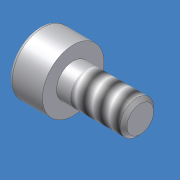
# Autodesk Inventor part: 520204172
Saved by Autodesk Inventor 2021.3 (Build 253353000, 353)
## iProperties
Manager: SRONS
Created: 2005-03-16
Part Number: 520204172
Material: Allgemein
Vendor: Autodesk Inc.
Document SubType Name: Modeling
Standard: DIN 912
Designer: SROAMA
Size Designation: M3 x 6
User Status: Zurückgezogen
Engineer: SROAMA
Density: 1 g/cm^3
Appearance: Vorgabe
Mass: 0.104143 g
Surface Area: 1.64552 cm^2
Volume: 0.104143 cm^3
Description: Zyl-Schr M3 x 6 DIN 912 A4 BN 612
Title: Zyl-Schr M3 x 6 DIN 912 A4 BN 612
Author: SROAMA
EGR: 1
Classification: un/spsc 31161501
Design Tracking - Titel: M3 x 6
Dateiname: 520_204_172
Zeichnungsummer: 520 204 172
Erstellt_am: 16.01.2008
Erstellt_durch: KC
Status: Veraltet
Titel: Zyl-Schr M3 x 6 ISO 4762 Inox A4
Zeichnungsname: 520 204 172
Zeichnungsnummer: 520204172
DOCID: 218911
PDB_IDENT: 520204172
PDB_Name: 520204172
PDB_Ident_Ver: =<PDB_Ident> <PDB_Version>
STID: 28675
ROT_Weight: 0.104 g
ROT_Weight_Num: 0.00010414301452605634
_DisabledCommands: 0
Autodesk Inventor part; units mm, degrees
ref_plane "YZ Plane" through (0, 0, 0) normal (1, 0, 0) x (0, 1, 0)
ref_plane "XZ Plane" through (0, 0, 0) normal (0, 1, 0) x (-1, 0, 0)
ref_plane "XY Plane" through (0, 0, 0) normal (0, 0, 1) x (1, 0, 0)
sketch "Skizze1" plane through (0, 0, 0) normal (0, 0, 1) x (1, 0, 0)
  line L0 (-0.8667, 0) -> (6, 0)
  line L1 (6, 0) -> (6, 1.5)
  line L2 (6, 1.5) -> (1.25, 1.5)
  line L3 (1.25, 1.5) -> (0.9432, 1.5)
  line L4 (0.9432, 1.5) -> (0, 1.5)
  line L5 (0, 1.5) -> (0, 2.75)
  line L6 (0, 2.75) -> (-3, 2.75)
  line L7 (-3, 2.75) -> (-3, 1.4434)
  line L8 (-3, 1.4434) -> (-1.7, 1.4434)
  line L9 (-1.7, 1.4434) -> (-0.8667, 0)
  line L10 (-15.5, 0) -> (61.5, 0) projected
  line L11 (0, -0.8) -> (0, 10.4) projected
  line L12 (1.25, 1.5) -> (0, 1.5) construction
  dimension "d1" = 4.75
  dimension "d2" = 0.3068
  dimension "d3" = 3
  dimension "d4" = 1.3
  dimension "d5" = 60
  dimension "d6" = 3
  dimension "d7" = 3
  dimension "d8" = 2.8868
  dimension "d9" = 5.5
  dimension "d26" = 6
  constraints: 22 end point, 6 parallel, 2 collinear, 2 perpendicular, 1 horizontal, 1 point on line
  measures "d1" distance from line of L2.end L1
  measures "d2" distance of L3.end L2.end
  measures "d3" distance between parallel lines of L7 L5
  measures "d4" distance of L7.end L8.end
  measures "d5" angle of L9 L0
  measures "d6" diameter of L2 L0
  measures "d7" diameter of L4 L0
  measures "d8" diameter of L8 L0
  measures "d9" diameter of L6 L0
  measures "d26" distance between parallel lines of L11 L1
revolve "Körper" add sketch "Skizze1" angle 360 about axis through (-0.8667, 0, 0) along (1, 0, 0)
sketch "Skizze2" plane through (-3, 0, 0) normal (-1, 0, 0) x (0, 0, 1)
  circle A0 centre (0, 0) radius 1.4434 projected
  line L0 (0, -3.3) -> (0, 4.4) projected
  line L1 (-3.3, 0) -> (4.4, 0) projected
  line L2 (1.4434, 0) -> (0.7217, -1.25)
  line L3 (0.7217, -1.25) -> (-0.7217, -1.25)
  line L4 (-0.7217, -1.25) -> (-1.4434, 0)
  line L5 (-1.4434, 0) -> (-0.7217, 1.25)
  line L6 (-0.7217, 1.25) -> (0.7217, 1.25)
  line L7 (0.7217, 1.25) -> (1.4434, 0)
  constraints: 12 end point, 1 coincident, 1 horizontal alignment, 1 point on line, 12 other
extrude "Loch" add sketch "Skizze2" against normal up to next contours L7 A0 | A0 L2 | L6 L0 A0 | A0 L0 L3 | L0 L6 A0 | A0 L3 L0 | L4 A0 | A0 L5
fillet "Rundung1" radius 0.3 1 edges at (-3, -2.75, 0)
thread "Gewinde" size "M3x0.5" designation "M3" class "6g" standard "ANSI Metrisches M Profil" length 4.75
chamfer "Fase1" distance 0.3067 distance2 0.3067 1 edges at (6, -1.5, 0) measured on face at (6, -0.2617, -0.7882)
equation "\"d1\" = GEL"
equation "\"d3\" = KOH"
equation "\"d4\" = INTI"
equation "\"d6\" = GD"
equation "\"d7\" = BDM"
equation "\"d8\" = 1.1547 * SW"
equation "\"d9\" = KOD"
equation "\"d26\" = NLG"
equation "\"d17\" = RR"
equation "\"d13\" = GEL"
equation "\"d15\" = -0.5 * SPD + 0.5 * GD"
equation "\"d16\" = GUL"
equation "\"GD\" = NND"
equation "\"NLG\" = 6"
equation "\"GEL\" = 4.75"
equation "\"KOD\" = 5.5"
equation "\"KOH\" = 3"
equation "\"INTI\" = 1.3"
equation "\"GAL\" = 0.61345 * TPU"
equation "\"GUL\" = 0.61345 * TPU"
equation "\"BDM\" = NND"
equation "\"SW\" = 2.5"
equation "\"RR\" = 0.1 * KOH"
equation "\"SPD\" = NND - 1.2269 * TPU"
equation "\"NND\" = 3"
equation "\"E0\" = 1.155 * SW"
equation "\"ANG\" = 120deg"
equation "\"FAWI\" = 45deg"
equation "\"THREADDIA\" = 3"
equation "\"TPU\" = 0.5"
equation "\"GD1\" = THREADDIA - 1.2269 * TPU"
equation "\"PTC\" = TPU"
equation "\"TOA\" = 30deg"
